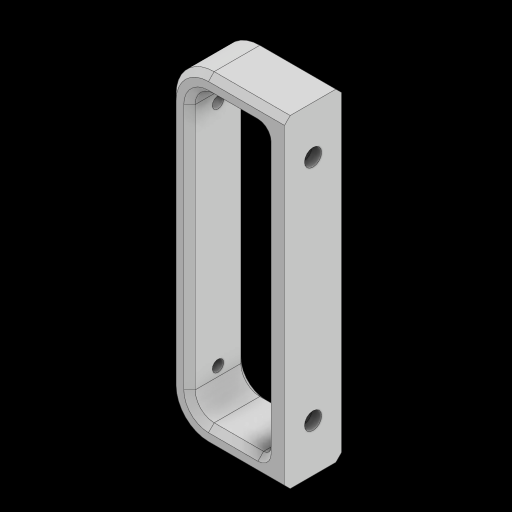
# Autodesk Inventor part: 260_Handle
Saved by Autodesk Inventor 2024 (Build 280153000, 153)
## iProperties
Created: 2023-07-27
Part Number: 260_Handle
Material: Generisch
Document SubType Name: Modeling
Designer: Philipp
Density: 1 g/cm^3
Appearance: Vorgabe
Author: Philipp
Autodesk Inventor part; units mm, degrees
ref_plane "YZ Plane" through (0, 0, 0) normal (1, 0, 0) x (0, 1, 0)
ref_plane "XZ Plane" through (0, 0, 0) normal (0, 1, 0) x (-1, 0, 0)
ref_plane "XY Plane" through (0, 0, 0) normal (0, 0, 1) x (1, 0, 0)
sketch "Skizze1" plane through (0, 0, 0) normal (0, 1, 0) x (-1, 0, 0)
  line L0 (0, 0) -> (5, 0)
  line L1 (5, 0) -> (5, -85)
  line L2 (5, -85) -> (0, -85)
  line L3 (0, -85) -> (0, 0)
  line L4 (0, 0) -> (25, 0)
  line L5 (25, 0) -> (25, -5)
  line L6 (25, -5) -> (0, -5)
  line L7 (0, -5) -> (0, 0)
  line L8 (25, 0) -> (30, 0)
  line L9 (30, 0) -> (30, -85)
  line L10 (30, -85) -> (25, -85)
  line L11 (25, -85) -> (25, 0)
  line L12 (30, -85) -> (0, -85)
  line L13 (0, -85) -> (0, -80)
  line L14 (0, -80) -> (30, -80)
  line L15 (30, -80) -> (30, -85)
  point P0 (5, -5)
  point P1 (25, -80)
  point P2 (5, -80)
  dimension "d0" = 5
  dimension "d1" = 85
  dimension "d2" = 25
  dimension "d3" = 5
  dimension "d4" = 5
  dimension "d5" = 85
  dimension "d13" = 30
  dimension "d14" = 5
  constraints: 32 end point, 8 parallel, 4 horizontal, 4 perpendicular
  measures "d0" distance of L1.end L2.end
  measures "d1" distance of L0.end L1.end
  measures "d2" distance of L5.end L6.end
  measures "d3" distance of L4.end L5.end
  measures "d4" distance of L9.end L10.end
  measures "d5" distance of L8.end L9.end
  measures "d13" distance of L13.end L14.end
  measures "d14" distance of L12.end L13.end
extrude "Extrusion1" add sketch "Skizze1" along normal blind 15 contours L0 L1 L6 L3 | L4 L5 L6 L1 | L6 L1 L14 L3 | L8 L9 L14 L11 L5 | L14 L1 L2 L3 | L14 L11 L12 L1 | L14 L9 L10 L11
fillet "Rundung1" radius 10 2 edges at (-30, 7.5, 0) (-30, 7.5, -85)
fillet "Rundung2" radius 5 2 edges at (-25, 7.5, -5) (-25, 7.5, -80)
fillet "Rundung3" radius 2 2 edges at (-5, 7.5, -5) (-5, 7.5, -80)
sketch "Skizze2" plane through (-5, 0, -75) normal (-1, 0, 0) x (0, 0, 1)
  line L0 (-10, 0) -> (-10, 15) projected
  line L1 (-10, 7.5) -> (75, 7.5) construction
  line L2 (75, 0) -> (75, 15) construction
  point P0 (62.5, 7.5)
  point P1 (2.5, 7.5)
  dimension "d15" = 60
  dimension "d16" = 12.5
  constraints: 2 end point, 2 midpoint, 2 point on line
  measures "d15" distance of point (2.5, 7.5) point (62.5, 7.5)
  measures "d16" distance of L1.start point (2.5, 7.5)
hole "Bohrung1" at (-5, 7.5, -12.5) at (-5, 7.5, -72.5) direction (1, 0, 0) diameter 4.5 depth 5 countersink diameter 9.4 countersink angle 90 clearance for "Flachkopfsenkschraube ISO 2009/7046" size "M4" standard "ISO"
sketch "Skizze3" plane through (-30, 0, -75) normal (-1, 0, 0) x (0, 0, 1)
  circle A0 centre (2.5, 7.5) radius 4.7 projected
  circle A1 centre (62.5, 7.5) radius 4.7 projected
  circle A2 centre (2.5, 7.5) radius 2.25 projected
  point P0 (75, 0)
  constraints: 2 coincident
hole "Bohrung2" at (-30, 7.5, -72.5) at (-30, 7.5, -12.5) direction (1, 0, 0) diameter 3 depth 25
chamfer "Fasen1" distance 1.5 angle 45 8 edges at (-5, 0, -42.5) (-13.5, 0, -5) (-25, 0, -42.5) (-13.5, 0, -80) (-5, 15, -42.5) (-13.5, 15, -5) (-25, 15, -42.5) (-13.5, 15, -80)
chamfer "Fasen2" distance 1.5 angle 45 10 edges at (-30, 0, -42.5) (-27.0711, 0, -2.9289) (-10, 0, 0) (-27.0711, 0, -82.0711) (-10, 0, -85) (-30, 15, -42.5) (-27.0711, 15, -2.9289) (-10, 15, 0) (-27.0711, 15, -82.0711) (-10, 15, -85)
